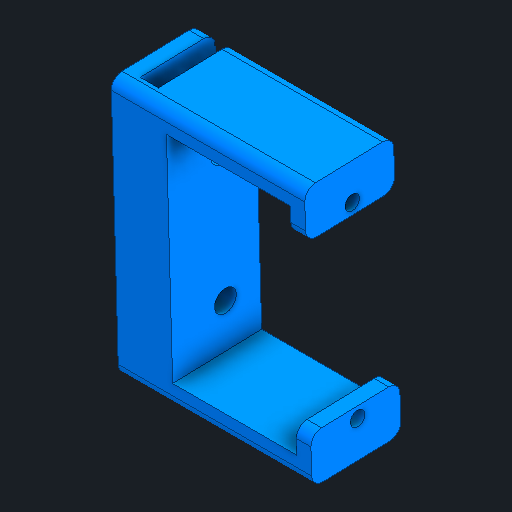
# Autodesk Inventor part: servo_mount
Saved by Autodesk Inventor 2023 (Build 270158030, 158C)
## iProperties
Created: 2022-03-29
Part Number: servo_mount
Material: Generic
Document SubType Name: Modeling
Designer: kardo
Density: 1 g/cm^3
Appearance: Blue Plastic
Author: kardo
Autodesk Inventor part; units mm, degrees
ref_plane "YZ Plane" through (0, 0, 0) normal (1, 0, 0) x (0, 1, 0)
ref_plane "XZ Plane" through (0, 0, 0) normal (0, 1, 0) x (-1, 0, 0)
ref_plane "XY Plane" through (0, 0, 0) normal (0, 0, 1) x (1, 0, 0)
derived "stencil_frame.ipt"
sketch "sk_servo_joint" plane through (-54.6, 0, 0) normal (1, 0, 0) x (0, 1, 0)
  line L0 (-254.1001, 21.0191) -> (9.48, 28.5282) construction
  line L1 (-363, 4666.1952) -> (-363, -2045.0469) construction
  line L2 (0, 4666.1952) -> (0, -2045.0469) construction
  line L3 (-204.8284, 22.4228) -> (-205.0163, 29.0201) construction
  line L4 (-205.0163, 29.0201) -> (-187.0237, 29.5327) construction
  line L5 (-187.0237, 29.5327) -> (-186.8357, 22.9354) construction
  line L6 (-96.0606, 32.1241) -> (-98.9083, 132.0836) construction
  line L7 (-98.9083, 132.0836) -> (-198.8678, 129.2358) construction
  line L8 (-198.8678, 129.2358) -> (-196.02, 29.2764) construction
  line L9 (-187.0237, 29.5327) -> (-96.0606, 32.1241) construction
  point P0 (0, 0)
  point P1 (-190.9494, 44.4269)
sketch3d "sk_servo_rod"
ref_plane "plane_cowl_left" through (-54.6, 0, 0) normal (1, 0, 0) x (0, 1, 0)
derived "parameters_frame.ipt"
derived "parameters_powertrain.ipt"
sketch "sk_base" plane through (-54.6, 0, 0) normal (1, 0, 0) x (0, 1, 0)
  line L0 (-254.1001, 21.0191) -> (9.48, 28.5282) construction
  line L1 (-210.8772, 24.0512) -> (-180.8894, 24.9055)
  line L2 (-180.8894, 24.9055) -> (-181.1799, 35.1014)
  line L3 (-181.1799, 35.1014) -> (-211.1677, 34.247)
  line L4 (-211.1677, 34.247) -> (-210.8772, 24.0512)
  line L5 (-205.0163, 29.0201) -> (-211.0139, 28.8492) construction
  line L6 (-187.0237, 29.5327) -> (-181.0261, 29.7036) construction
  line L7 (-210.8772, 24.0512) -> (-213.876, 23.9657)
  line L8 (-213.876, 23.9657) -> (-214.2234, 36.1608)
  line L9 (-214.2234, 36.1608) -> (-178.238, 37.186)
  line L10 (-178.238, 37.186) -> (-177.8906, 24.9909)
  line L11 (-177.8906, 24.9909) -> (-180.8894, 24.9055)
  point P0 (0, 0)
  point P1 (-196.02, 29.2764)
  dimension "d1" = 18
  dimension "d2" = 1.8
  dimension "d5" = 5.4
  dimension "d6" = 30
  dimension "d8" = 2
  dimension "d9" = 3
  constraints: 22 end point, 5 parallel, 4 collinear, 4 perpendicular, 2 point on line
  measures "d1" distance of L6.start L5.start
  measures "d2" distance between parallel lines of L0 L1
  measures "d5" distance from line of point (-196.02, 29.276) L3
  measures "d6" distance between parallel lines of L2 L4
  measures "d8" distance between parallel lines of L9 L3
  measures "d9" distance between parallel lines of L8 L4
sketch "sk_side_rails" plane through (-54.6, 0, 0) normal (1, 0, 0) x (0, 1, 0)
  line L0 (-211.1677, 34.247) -> (-210.8772, 24.0512) projected
  line L1 (-180.8894, 24.9055) -> (-181.1799, 35.1014) projected
  line L2 (-213.876, 23.9657) -> (-210.8772, 24.0512)
  line L3 (-177.8906, 24.9909) -> (-180.8894, 24.9055)
  line L4 (-214.2234, 36.1608) -> (-178.238, 37.186) projected
  line L5 (-213.876, 23.9657) -> (-214.2234, 36.1608) projected
  line L6 (-178.238, 37.186) -> (-177.8906, 24.9909) projected
  line L7 (-210.8772, 24.0512) -> (-213.876, 23.9657) projected
  line L8 (-177.8906, 24.9909) -> (-180.8894, 24.9055) projected
  line L9 (-211.1677, 34.247) -> (-211.2247, 36.2462)
  line L10 (-181.1799, 35.1014) -> (-181.2368, 37.1006)
  point P0 (0, 0)
  constraints: 8 end point, 2 collinear, 2 perpendicular, 2 point on line
sketch "sk_bridge" plane through (-54.6, 0, 0) normal (1, 0, 0) x (0, 1, 0)
  line L0 (-214.2234, 36.1608) -> (-178.238, 37.186) projected
  line L1 (-181.1799, 35.1014) -> (-211.1677, 34.247) projected
  line L2 (-214.2234, 36.1608) -> (-214.1665, 34.1616)
  line L3 (-214.1665, 34.1616) -> (-211.1677, 34.247)
  line L4 (-178.238, 37.186) -> (-178.1811, 35.1868)
  line L5 (-178.1811, 35.1868) -> (-181.1799, 35.1014)
  point P0 (0, 0)
  constraints: 8 end point, 2 collinear, 2 perpendicular
extrude "extrude_bridge" add sketch "sk_bridge" against normal blind 2.5
extrude "extrude_rails" add sketch "sk_side_rails" along normal blind 22
sketch "sk_backplate" plane through (-57.1, 0, 0) normal (-1, 0, 0) x (0, 0, 1)
  line L0 (37.186, -178.238) -> (24.9909, -177.8906) projected
  line L1 (24.0512, -210.8772) -> (24.9055, -180.8894) projected
  line L2 (24.9909, -177.8906) -> (24.9055, -180.8894) projected
  line L3 (24.0512, -210.8772) -> (23.9657, -213.876) projected
  line L4 (23.9657, -213.876) -> (36.1608, -214.2234) projected
  line L5 (36.1608, -214.2234) -> (37.186, -178.238) projected
  point P0 (0, 0)
extrude "extrude_backplate" add sketch "sk_backplate" along normal blind 2
sketch "sk_frontplate" plane through (-54.6, 0, 0) normal (1, 0, 0) x (0, 1, 0)
  line L0 (-213.876, 23.9657) -> (-214.2234, 36.1608) projected
  line L1 (-214.2234, 36.1608) -> (-178.238, 37.186) projected
  line L2 (-178.238, 37.186) -> (-177.8906, 24.9909) projected
  line L3 (-177.8906, 24.9909) -> (-180.8894, 24.9055) projected
  line L4 (-210.8772, 24.0512) -> (-180.8894, 24.9055) projected
  line L5 (-210.8772, 24.0512) -> (-213.876, 23.9657) projected
  point P0 (0, 0)
extrude "extrude_frontplate" add sketch "sk_frontplate" along normal blind 3
sketch "sk_drills" plane through (-54.6, 0, 0) normal (1, 0, 0) x (0, 1, 0)
  line L0 (-205.0163, 29.0201) -> (-187.0237, 29.5327) construction
  line L1 (-203.3534, 32.0998) -> (-201.5178, 29.1198)
  line L2 (-201.5178, 29.1198) -> (-203.1807, 26.0401)
  line L3 (-203.1807, 26.0401) -> (-206.6793, 25.9404)
  line L4 (-206.6793, 25.9404) -> (-208.5149, 28.9204)
  line L5 (-208.5149, 28.9204) -> (-206.852, 32.0001)
  line L6 (-206.852, 32.0001) -> (-203.3534, 32.0998)
  line L7 (-185.3607, 32.6124) -> (-183.5251, 29.6324)
  line L8 (-183.5251, 29.6324) -> (-185.188, 26.5527)
  line L9 (-185.188, 26.5527) -> (-188.6866, 26.453)
  line L10 (-188.6866, 26.453) -> (-190.5222, 29.433)
  line L11 (-190.5222, 29.433) -> (-188.8593, 32.5127)
  line L12 (-188.8593, 32.5127) -> (-185.3607, 32.6124)
  circle A0 centre (-205.0163, 29.0201) radius 1.5
  circle A1 centre (-187.0237, 29.5327) radius 1.5
  point P0 (0, 0)
  dimension "d19" = 7
  dimension "d20" = 3
  constraints: 26 end point, 4 coincident, 2 centre point, 2 point on line, 1 collinear, 1 equal radius, 26 other
  measures "d19" distance of L1.end L4.end
  measures "d20" diameter of A1
extrude "drill_hex_backplate" cut sketch "sk_drills" against normal through all contours L1 L2 L3 L4 L5 L6 | L7 L8 L9 L10 L11 L12 | A0 | A1
extrude "drill_circular_frontplate" cut sketch "sk_drills" along normal through all contours A0 | A1
sketch "sk_mounting_pads" plane through (-32.6, 0, 0) normal (1, 0, 0) x (0, 0, -1)
  line L0 (-24.0512, -210.8772) -> (-36.2462, -211.2247) projected
  line L1 (-37.1006, -181.2368) -> (-24.9055, -180.8894) projected
  line L2 (-36.2462, -211.2247) -> (-36.3459, -207.7261)
  line L3 (-36.3459, -207.7261) -> (-24.1508, -207.3786)
  line L4 (-24.1508, -207.3786) -> (-24.0512, -210.8772)
  line L5 (-37.1006, -181.2368) -> (-37.0009, -184.7354)
  line L6 (-37.0009, -184.7354) -> (-24.8058, -184.388)
  line L7 (-24.8058, -184.388) -> (-24.9055, -180.8894)
  point P0 (0, 0)
  dimension "d37" = 23
  constraints: 12 end point, 4 perpendicular, 2 parallel, 1 collinear
  measures "d37" distance between parallel lines of L6 L3
extrude "extrude_mounting_pads" add sketch "sk_mounting_pads" against normal blind 2
sketch "sk_pad_drills" plane through (-32.6, 0, 0) normal (1, 0, 0) x (0, 0, -1)
  line L0 (-24.1508, -207.3786) -> (-36.3459, -207.7261) construction
  line L1 (-37.0009, -184.7354) -> (-24.8058, -184.388) construction
  line L2 (-29.9058, -209.0432) -> (-29.9485, -207.5438) construction
  line L3 (-30.6035, -184.5531) -> (-30.6462, -183.0537) construction
  line L4 (-29.9485, -207.5438) -> (-30.6035, -184.5531) construction
  line L5 (-29.0201, -205.0163) -> (-128.9795, -207.8641) construction
  line L6 (-128.9795, -207.8641) -> (-129.4921, -189.8714) construction
  line L7 (-129.4921, -189.8714) -> (-29.5327, -187.0237) construction
  circle A0 centre (-29.0201, -205.0163) radius 1.5 projected
  line L8 (-29.5327, -187.0237) -> (-29.0201, -205.0163) construction
  point P0 (0, 0)
  dimension "d39" = 26
  dimension "d40" = 100
  dimension "d41" = 99
  constraints: 14 end point, 3 collinear, 2 parallel, 2 perpendicular, 2 point on line
  measures "d39" distance of L2.start L3.end
  measures "d40" distance of L5.start L5.end
  measures "d41" distance between parallel lines of L6 L4
hole "drill_pads" at (-32.6, -209.0432, 29.9058) at (-32.6, -183.0537, 30.6462) direction (-1, 0, 0) diameter 2 depth 2 tip angle 118
fillet "rounding" radius 1.5 10 edges at (-45.85, -178.238, 37.186) (-43.6, -177.8906, 24.9909) (-58.1, -177.8906, 24.9909) (-43.6, -213.876, 23.9657) (-45.85, -214.2234, 36.1608) (-58.1, -213.876, 23.9657) (-33.6, -207.7261, 36.3459) (-33.6, -207.3786, 24.1508) (-33.6, -184.7354, 37.0009) (-33.6, -184.388, 24.8058)
equation "\"d5\" = 1.8 * drill_servo_mount_diam"
equation "\"d12\" = servo_pad_height_gross"
equation "\"d20\" = drill_servo_mount_diam"
equation "\"d39\" = servo_width + 2 * servo_pad_drill_outset"
equation "\"d41\" = d40 - servo_pad_drill_centerline"
equation "\"d30\" = servo_pad_drill_diam"
equation "\"servo_pad_height_gross\" = 22"
equation "\"drill_servo_mount_diam\" = 3"
equation "\"servo_width\" = 22"
equation "\"servo_pad_drill_outset\" = 2"
equation "\"servo_pad_drill_centerline\" = 1"
equation "\"servo_pad_drill_diam\" = 2"
body "Solid1"
